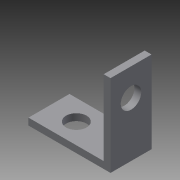
# Autodesk Inventor part: LBlock
Saved by Autodesk Inventor 2016 (Build 200138000, 138)
## iProperties
Created: 2016-04-07
Part Number: LBlock
Material: Generic
Document SubType Name: Modeling
Designer: Ethan
Density: 1 g/cm^3
Appearance: Default
Author: Ethan
Autodesk Inventor part; units mm, degrees
ref_plane "YZ Plane" through (0, 0, 0) normal (1, 0, 0) x (0, 1, 0)
ref_plane "XZ Plane" through (0, 0, 0) normal (0, 1, 0) x (-1, 0, 0)
ref_plane "XY Plane" through (0, 0, 0) normal (0, 0, 1) x (1, 0, 0)
sketch "Sketch1" plane through (0, 0, 0) normal (0, 1, 0) x (-1, 0, 0)
  line L0 (8.6591, 4.7625) -> (-10.3909, 4.7625)
  line L1 (-10.3909, 4.7625) -> (-10.3909, -4.7625)
  line L2 (-10.3909, -4.7625) -> (8.6591, -4.7625)
  line L3 (8.6591, -4.7625) -> (8.6591, 4.7625)
  circle A0 centre (2.3091, 0) radius 2.3813
  line L4 (-10.3909, 4.7625) -> (-8.8034, 4.7625)
  line L5 (-8.8034, 4.7625) -> (-8.8034, -4.7625)
  line L6 (-8.8034, -4.7625) -> (-10.3909, -4.7625)
  line L7 (-10.3909, -4.7625) -> (-10.3909, 4.7625)
  point P0 (0, 0)
  dimension "d0" = 19.05
  dimension "d1" = 9.525
  dimension "d3" = 4.7625
  dimension "d4" = 12.7
  dimension "d5" = 1.5875
  constraints: 16 end point, 4 parallel, 2 horizontal, 2 perpendicular, 1 centre point, 1 point on line
  measures "d0" distance of L0.start L0.end
  measures "d1" distance of L2.end L0.start
  measures "d3" diameter of A0
  measures "d4" distance from line of L1 A0.centre
  measures "d5" distance between parallel lines of L1 L5
extrude "Extrusion1" add sketch "Sketch1" along normal blind 1.5875 contours L3 L2 L5 L0
extrude "Extrusion2" add sketch "Sketch1" along normal blind 19.05 contours L5 L2 L1 L0
sketch "Sketch2" plane through (10.3909, 0, 4.7625) normal (1, 0, 0) x (0, 0, -1)
  circle A0 centre (4.7625, 12.7) radius 2.3813
  point P0 (4.7625, 0)
  dimension "d10" = 12.7
  dimension "d11" = 4.7625
  constraints: 1 centre point
  measures "d10" distance of point (4.762, 0) A0.centre
  measures "d11" diameter of A0
extrude "Extrusion3" cut sketch "Sketch2" against normal blind 1.5875
body "Solid1"
